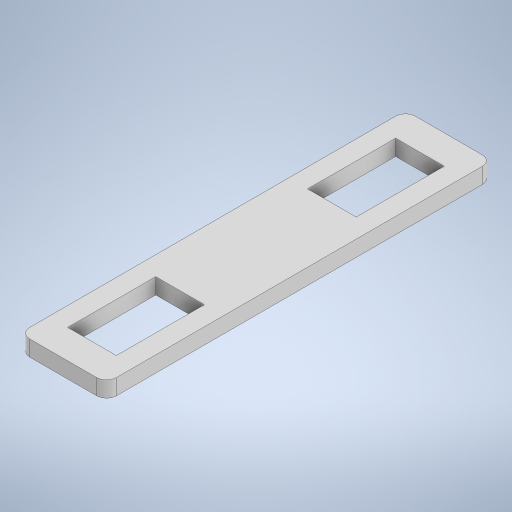
# Autodesk Inventor part: arm_medium_part_v2
Saved by Autodesk Inventor 2023 (Build 270158000, 158)
## iProperties
Created: 2023-02-22
Part Number: arm_medium_part_v2
Material: Ogólny
Document SubType Name: Modeling
Designer: kamil
Density: 1 g/cm^3
Appearance: Domyślna
Author: kamil
Autodesk Inventor part; units mm, degrees
ref_plane "YZ Plane" through (0, 0, 0) normal (1, 0, 0) x (0, 1, 0)
ref_plane "XZ Plane" through (0, 0, 0) normal (0, 1, 0) x (-1, 0, 0)
ref_plane "XY Plane" through (0, 0, 0) normal (0, 0, 1) x (1, 0, 0)
sketch "Szkic1" plane through (0, 0, 0) normal (0, 1, 0) x (-1, 0, 0)
  line L0 (8.75, 50) -> (-8.75, 50)
  line L1 (-11.25, 47.5) -> (-11.25, -47.5)
  line L2 (-8.75, -50) -> (8.75, -50)
  line L3 (11.25, -47.5) -> (11.25, 47.5)
  line L4 (-11.25, 50) -> (11.25, -50)
  line L5 (-11.25, -50) -> (11.25, 50)
  arc A0 (11.25, 47.5) -> (8.75, 50) centre (8.75, 47.5) ccw
  arc A1 (-8.75, 50) -> (-11.25, 47.5) centre (-8.75, 47.5) ccw
  arc A2 (-11.25, -47.5) -> (-8.75, -50) centre (-8.75, -47.5) ccw
  arc A3 (8.75, -50) -> (11.25, -47.5) centre (8.75, -47.5) ccw
  point P0 (0, 0)
  point P1 (0, 0)
  dimension "d0" = 22.5
  dimension "d1" = 100
  dimension "d2" = 2.5
  constraints: 12 end point, 8 point on circle, 8 point on line, 8 tangent, 4 centre point, 3 equal radius, 2 parallel, 1 coincident, 1 horizontal, 1 midpoint, 1 perpendicular
  measures "d0" distance of L4.end L5.start
  measures "d1" distance of L5.start L4.start
  measures "d2" radius of A0
extrude "Wyciągnięcie proste1" add sketch "Szkic1" along normal blind 4.1
sketch "Szkic2" plane through (0, 4.1, 0) normal (0, 1, 0) x (1, 0, 0)
  line L0 (-6.3, -42.5) -> (6.3, -42.5)
  line L1 (6.3, -42.5) -> (6.3, -19.7)
  line L2 (6.3, -19.7) -> (-6.3, -19.7)
  line L3 (-6.3, -19.7) -> (-6.3, -42.5)
  line L4 (-8.75, -50) -> (8.75, -50) projected
  line L5 (11.25, -47.5) -> (11.25, 47.5) projected
  line L6 (-6.3, 19.7) -> (6.3, 19.7)
  line L7 (6.3, 19.7) -> (6.3, 42.5)
  line L8 (6.3, 42.5) -> (-6.3, 42.5)
  line L9 (-6.3, 42.5) -> (-6.3, 19.7)
  line L10 (-15.75, 0) -> (15.75, 0) projected
  point P0 (0, 0)
  point P1 (0, -42.5)
  dimension "d5" = 12.6
  dimension "d6" = 22.8
  dimension "d7" = 7.5
  dimension "d8" = 11.25
  constraints: 16 end point, 4 parallel, 2 equal length, 2 horizontal, 2 perpendicular, 1 midpoint, 2 other
  measures "d5" distance of L2.end L1.end
  measures "d6" distance of L1.end L0.end
  measures "d7" distance between parallel lines of L4 L0
  measures "d8" distance from line of L5 point (0, -42.5)
extrude "Wyciągnięcie proste2" cut sketch "Szkic2" against normal blind 4.1
